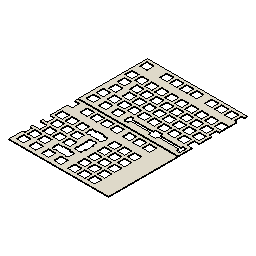
plate - F3D (Autodesk Fusion 360 design; units mm, degrees)
Autodesk Fusion 360 part; units mm, degrees
note: some values were not read from the file. Chosen so that the rebuilt part matches the saved one: which bodies a step acts on.
(part 1 of 3)
sketch "plate-2026-02-23T17_51_34.543Z" plane through (0, 0, 0) normal (0, 1, 0) x (1, 0, 0)
  line L0 (3.025, -2.525) -> (16.025, -2.525)
  line L1 (3.025, -16.525) -> (16.025, -16.525)
  line L2 (2.525, -3.025) -> (2.525, -16.025)
  line L3 (16.525, -3.025) -> (16.525, -16.025)
  arc A0 (3.025, -2.525) -> (2.525, -3.025) centre (3.025, -3.025) ccw
  arc A1 (16.525, -3.025) -> (16.025, -2.525) centre (16.025, -3.025) ccw
  arc A2 (2.525, -16.025) -> (3.025, -16.525) centre (3.025, -16.025) ccw
  arc A3 (16.025, -16.525) -> (16.525, -16.025) centre (16.025, -16.025) ccw
  line L4 (41.125, -2.525) -> (54.125, -2.525)
  line L5 (41.125, -16.525) -> (54.125, -16.525)
  line L6 (40.625, -3.025) -> (40.625, -16.025)
  line L7 (54.625, -3.025) -> (54.625, -16.025)
  arc A4 (41.125, -2.525) -> (40.625, -3.025) centre (41.125, -3.025) ccw
  arc A5 (54.625, -3.025) -> (54.125, -2.525) centre (54.125, -3.025) ccw
  arc A6 (40.625, -16.025) -> (41.125, -16.525) centre (41.125, -16.025) ccw
  arc A7 (54.125, -16.525) -> (54.625, -16.025) centre (54.125, -16.025) ccw
  line L8 (60.175, -2.525) -> (73.175, -2.525)
  line L9 (60.175, -16.525) -> (73.175, -16.525)
  line L10 (59.675, -3.025) -> (59.675, -16.025)
  line L11 (73.675, -3.025) -> (73.675, -16.025)
  arc A8 (60.175, -2.525) -> (59.675, -3.025) centre (60.175, -3.025) ccw
  arc A9 (73.675, -3.025) -> (73.175, -2.525) centre (73.175, -3.025) ccw
  arc A10 (59.675, -16.025) -> (60.175, -16.525) centre (60.175, -16.025) ccw
  arc A11 (73.175, -16.525) -> (73.675, -16.025) centre (73.175, -16.025) ccw
  line L12 (79.225, -2.525) -> (92.225, -2.525)
  line L13 (79.225, -16.525) -> (92.225, -16.525)
  line L14 (78.725, -3.025) -> (78.725, -16.025)
  line L15 (92.725, -3.025) -> (92.725, -16.025)
  arc A12 (79.225, -2.525) -> (78.725, -3.025) centre (79.225, -3.025) ccw
  arc A13 (92.725, -3.025) -> (92.225, -2.525) centre (92.225, -3.025) ccw
  arc A14 (78.725, -16.025) -> (79.225, -16.525) centre (79.225, -16.025) ccw
  arc A15 (92.225, -16.525) -> (92.725, -16.025) centre (92.225, -16.025) ccw
  line L16 (98.275, -2.525) -> (111.275, -2.525)
  line L17 (98.275, -16.525) -> (111.275, -16.525)
  line L18 (97.775, -3.025) -> (97.775, -16.025)
  line L19 (111.775, -3.025) -> (111.775, -16.025)
  arc A16 (98.275, -2.525) -> (97.775, -3.025) centre (98.275, -3.025) ccw
  arc A17 (111.775, -3.025) -> (111.275, -2.525) centre (111.275, -3.025) ccw
  arc A18 (97.775, -16.025) -> (98.275, -16.525) centre (98.275, -16.025) ccw
  arc A19 (111.275, -16.525) -> (111.775, -16.025) centre (111.275, -16.025) ccw
  line L20 (126.85, -2.525) -> (139.85, -2.525)
  line L21 (126.85, -16.525) -> (139.85, -16.525)
  line L22 (126.35, -3.025) -> (126.35, -16.025)
  line L23 (140.35, -3.025) -> (140.35, -16.025)
  arc A20 (126.85, -2.525) -> (126.35, -3.025) centre (126.85, -3.025) ccw
  arc A21 (140.35, -3.025) -> (139.85, -2.525) centre (139.85, -3.025) ccw
  arc A22 (126.35, -16.025) -> (126.85, -16.525) centre (126.85, -16.025) ccw
  arc A23 (139.85, -16.525) -> (140.35, -16.025) centre (139.85, -16.025) ccw
  line L24 (145.9, -2.525) -> (158.9, -2.525)
  line L25 (145.9, -16.525) -> (158.9, -16.525)
  line L26 (145.4, -3.025) -> (145.4, -16.025)
  line L27 (159.4, -3.025) -> (159.4, -16.025)
  arc A24 (145.9, -2.525) -> (145.4, -3.025) centre (145.9, -3.025) ccw
  arc A25 (159.4, -3.025) -> (158.9, -2.525) centre (158.9, -3.025) ccw
  arc A26 (145.4, -16.025) -> (145.9, -16.525) centre (145.9, -16.025) ccw
  arc A27 (158.9, -16.525) -> (159.4, -16.025) centre (158.9, -16.025) ccw
  line L28 (164.95, -2.525) -> (177.95, -2.525)
  line L29 (164.95, -16.525) -> (177.95, -16.525)
  line L30 (164.45, -3.025) -> (164.45, -16.025)
  line L31 (178.45, -3.025) -> (178.45, -16.025)
  arc A28 (164.95, -2.525) -> (164.45, -3.025) centre (164.95, -3.025) ccw
  arc A29 (178.45, -3.025) -> (177.95, -2.525) centre (177.95, -3.025) ccw
  arc A30 (164.45, -16.025) -> (164.95, -16.525) centre (164.95, -16.025) ccw
  arc A31 (177.95, -16.525) -> (178.45, -16.025) centre (177.95, -16.025) ccw
  line L32 (184, -2.525) -> (197, -2.525)
  line L33 (184, -16.525) -> (197, -16.525)
  line L34 (183.5, -3.025) -> (183.5, -16.025)
  line L35 (197.5, -3.025) -> (197.5, -16.025)
  arc A32 (184, -2.525) -> (183.5, -3.025) centre (184, -3.025) ccw
  arc A33 (197.5, -3.025) -> (197, -2.525) centre (197, -3.025) ccw
  arc A34 (183.5, -16.025) -> (184, -16.525) centre (184, -16.025) ccw
  arc A35 (197, -16.525) -> (197.5, -16.025) centre (197, -16.025) ccw
  line L36 (212.575, -2.525) -> (225.575, -2.525)
  line L37 (212.575, -16.525) -> (225.575, -16.525)
  line L38 (212.075, -3.025) -> (212.075, -16.025)
  line L39 (226.075, -3.025) -> (226.075, -16.025)
  arc A36 (212.575, -2.525) -> (212.075, -3.025) centre (212.575, -3.025) ccw
  arc A37 (226.075, -3.025) -> (225.575, -2.525) centre (225.575, -3.025) ccw
  arc A38 (212.075, -16.025) -> (212.575, -16.525) centre (212.575, -16.025) ccw
  arc A39 (225.575, -16.525) -> (226.075, -16.025) centre (225.575, -16.025) ccw
  line L40 (231.625, -2.525) -> (244.625, -2.525)
  line L41 (231.625, -16.525) -> (244.625, -16.525)
  line L42 (231.125, -3.025) -> (231.125, -16.025)
  line L43 (245.125, -3.025) -> (245.125, -16.025)
  arc A40 (231.625, -2.525) -> (231.125, -3.025) centre (231.625, -3.025) ccw
  arc A41 (245.125, -3.025) -> (244.625, -2.525) centre (244.625, -3.025) ccw
  arc A42 (231.125, -16.025) -> (231.625, -16.525) centre (231.625, -16.025) ccw
  arc A43 (244.625, -16.525) -> (245.125, -16.025) centre (244.625, -16.025) ccw
  line L44 (250.675, -2.525) -> (263.675, -2.525)
  line L45 (250.675, -16.525) -> (263.675, -16.525)
  line L46 (250.175, -3.025) -> (250.175, -16.025)
  line L47 (264.175, -3.025) -> (264.175, -16.025)
  arc A44 (250.675, -2.525) -> (250.175, -3.025) centre (250.675, -3.025) ccw
  arc A45 (264.175, -3.025) -> (263.675, -2.525) centre (263.675, -3.025) ccw
  arc A46 (250.175, -16.025) -> (250.675, -16.525) centre (250.675, -16.025) ccw
  arc A47 (263.675, -16.525) -> (264.175, -16.025) centre (263.675, -16.025) ccw
  line L48 (269.725, -2.525) -> (282.725, -2.525)
  line L49 (269.725, -16.525) -> (282.725, -16.525)
  line L50 (269.225, -3.025) -> (269.225, -16.025)
  line L51 (283.225, -3.025) -> (283.225, -16.025)
  arc A48 (269.725, -2.525) -> (269.225, -3.025) centre (269.725, -3.025) ccw
  arc A49 (283.225, -3.025) -> (282.725, -2.525) centre (282.725, -3.025) ccw
  arc A50 (269.225, -16.025) -> (269.725, -16.525) centre (269.725, -16.025) ccw
  arc A51 (282.725, -16.525) -> (283.225, -16.025) centre (282.725, -16.025) ccw
  line L52 (293.5375, -2.525) -> (306.5375, -2.525)
  line L53 (293.5375, -16.525) -> (306.5375, -16.525)
  line L54 (293.0375, -3.025) -> (293.0375, -16.025)
  line L55 (307.0375, -3.025) -> (307.0375, -16.025)
  arc A52 (293.5375, -2.525) -> (293.0375, -3.025) centre (293.5375, -3.025) ccw
  arc A53 (307.0375, -3.025) -> (306.5375, -2.525) centre (306.5375, -3.025) ccw
  arc A54 (293.0375, -16.025) -> (293.5375, -16.525) centre (293.5375, -16.025) ccw
  arc A55 (306.5375, -16.525) -> (307.0375, -16.025) centre (306.5375, -16.025) ccw
  line L56 (312.5875, -2.525) -> (325.5875, -2.525)
  line L57 (312.5875, -16.525) -> (325.5875, -16.525)
  line L58 (312.0875, -3.025) -> (312.0875, -16.025)
  line L59 (326.0875, -3.025) -> (326.0875, -16.025)
  arc A56 (312.5875, -2.525) -> (312.0875, -3.025) centre (312.5875, -3.025) ccw
  arc A57 (326.0875, -3.025) -> (325.5875, -2.525) centre (325.5875, -3.025) ccw
  arc A58 (312.0875, -16.025) -> (312.5875, -16.525) centre (312.5875, -16.025) ccw
  arc A59 (325.5875, -16.525) -> (326.0875, -16.025) centre (325.5875, -16.025) ccw
  line L60 (331.6375, -2.525) -> (344.6375, -2.525)
  line L61 (331.6375, -16.525) -> (344.6375, -16.525)
  line L62 (331.1375, -3.025) -> (331.1375, -16.025)
  line L63 (345.1375, -3.025) -> (345.1375, -16.025)
  arc A60 (331.6375, -2.525) -> (331.1375, -3.025) centre (331.6375, -3.025) ccw
  arc A61 (345.1375, -3.025) -> (344.6375, -2.525) centre (344.6375, -3.025) ccw
  arc A62 (331.1375, -16.025) -> (331.6375, -16.525) centre (331.6375, -16.025) ccw
  arc A63 (344.6375, -16.525) -> (345.1375, -16.025) centre (344.6375, -16.025) ccw
  line L64 (3.025, -31.1) -> (16.025, -31.1)
  line L65 (3.025, -45.1) -> (16.025, -45.1)
  line L66 (2.525, -31.6) -> (2.525, -44.6)
  line L67 (16.525, -31.6) -> (16.525, -44.6)
  arc A64 (3.025, -31.1) -> (2.525, -31.6) centre (3.025, -31.6) ccw
  arc A65 (16.525, -31.6) -> (16.025, -31.1) centre (16.025, -31.6) ccw
  arc A66 (2.525, -44.6) -> (3.025, -45.1) centre (3.025, -44.6) ccw
  arc A67 (16.025, -45.1) -> (16.525, -44.6) centre (16.025, -44.6) ccw
  line L68 (22.075, -31.1) -> (35.075, -31.1)
  line L69 (22.075, -45.1) -> (35.075, -45.1)
  line L70 (21.575, -31.6) -> (21.575, -44.6)
  line L71 (35.575, -31.6) -> (35.575, -44.6)
  arc A68 (22.075, -31.1) -> (21.575, -31.6) centre (22.075, -31.6) ccw
  arc A69 (35.575, -31.6) -> (35.075, -31.1) centre (35.075, -31.6) ccw
  arc A70 (21.575, -44.6) -> (22.075, -45.1) centre (22.075, -44.6) ccw
  arc A71 (35.075, -45.1) -> (35.575, -44.6) centre (35.075, -44.6) ccw
  line L72 (41.125, -31.1) -> (54.125, -31.1)
  line L73 (41.125, -45.1) -> (54.125, -45.1)
  line L74 (40.625, -31.6) -> (40.625, -44.6)
  line L75 (54.625, -31.6) -> (54.625, -44.6)
  arc A72 (41.125, -31.1) -> (40.625, -31.6) centre (41.125, -31.6) ccw
  arc A73 (54.625, -31.6) -> (54.125, -31.1) centre (54.125, -31.6) ccw
  arc A74 (40.625, -44.6) -> (41.125, -45.1) centre (41.125, -44.6) ccw
  arc A75 (54.125, -45.1) -> (54.625, -44.6) centre (54.125, -44.6) ccw
  line L76 (60.175, -31.1) -> (73.175, -31.1)
  line L77 (60.175, -45.1) -> (73.175, -45.1)
  line L78 (59.675, -31.6) -> (59.675, -44.6)
  line L79 (73.675, -31.6) -> (73.675, -44.6)
  arc A76 (60.175, -31.1) -> (59.675, -31.6) centre (60.175, -31.6) ccw
  arc A77 (73.675, -31.6) -> (73.175, -31.1) centre (73.175, -31.6) ccw
  arc A78 (59.675, -44.6) -> (60.175, -45.1) centre (60.175, -44.6) ccw
  arc A79 (73.175, -45.1) -> (73.675, -44.6) centre (73.175, -44.6) ccw
  line L80 (79.225, -31.1) -> (92.225, -31.1)
  line L81 (79.225, -45.1) -> (92.225, -45.1)
  line L82 (78.725, -31.6) -> (78.725, -44.6)
  line L83 (92.725, -31.6) -> (92.725, -44.6)
  arc A80 (79.225, -31.1) -> (78.725, -31.6) centre (79.225, -31.6) ccw
  arc A81 (92.725, -31.6) -> (92.225, -31.1) centre (92.225, -31.6) ccw
  arc A82 (78.725, -44.6) -> (79.225, -45.1) centre (79.225, -44.6) ccw
  arc A83 (92.225, -45.1) -> (92.725, -44.6) centre (92.225, -44.6) ccw
  line L84 (98.275, -31.1) -> (111.275, -31.1)
  line L85 (98.275, -45.1) -> (111.275, -45.1)
  line L86 (97.775, -31.6) -> (97.775, -44.6)
  line L87 (111.775, -31.6) -> (111.775, -44.6)
  arc A84 (98.275, -31.1) -> (97.775, -31.6) centre (98.275, -31.6) ccw
  arc A85 (111.775, -31.6) -> (111.275, -31.1) centre (111.275, -31.6) ccw
  arc A86 (97.775, -44.6) -> (98.275, -45.1) centre (98.275, -44.6) ccw
  arc A87 (111.275, -45.1) -> (111.775, -44.6) centre (111.275, -44.6) ccw
  line L88 (117.325, -31.1) -> (130.325, -31.1)
  line L89 (117.325, -45.1) -> (130.325, -45.1)
  line L90 (116.825, -31.6) -> (116.825, -44.6)
  line L91 (130.825, -31.6) -> (130.825, -44.6)
  arc A88 (117.325, -31.1) -> (116.825, -31.6) centre (117.325, -31.6) ccw
  arc A89 (130.825, -31.6) -> (130.325, -31.1) centre (130.325, -31.6) ccw
  arc A90 (116.825, -44.6) -> (117.325, -45.1) centre (117.325, -44.6) ccw
  arc A91 (130.325, -45.1) -> (130.825, -44.6) centre (130.325, -44.6) ccw
  line L92 (136.375, -31.1) -> (149.375, -31.1)
  line L93 (136.375, -45.1) -> (149.375, -45.1)
  line L94 (135.875, -31.6) -> (135.875, -44.6)
  line L95 (149.875, -31.6) -> (149.875, -44.6)
  arc A92 (136.375, -31.1) -> (135.875, -31.6) centre (136.375, -31.6) ccw
  arc A93 (149.875, -31.6) -> (149.375, -31.1) centre (149.375, -31.6) ccw
  arc A94 (135.875, -44.6) -> (136.375, -45.1) centre (136.375, -44.6) ccw
  arc A95 (149.375, -45.1) -> (149.875, -44.6) centre (149.375, -44.6) ccw
  line L96 (155.425, -31.1) -> (168.425, -31.1)
  line L97 (155.425, -45.1) -> (168.425, -45.1)
  line L98 (154.925, -31.6) -> (154.925, -44.6)
  line L99 (168.925, -31.6) -> (168.925, -44.6)
  arc A96 (155.425, -31.1) -> (154.925, -31.6) centre (155.425, -31.6) ccw
  arc A97 (168.925, -31.6) -> (168.425, -31.1) centre (168.425, -31.6) ccw
  arc A98 (154.925, -44.6) -> (155.425, -45.1) centre (155.425, -44.6) ccw
  arc A99 (168.425, -45.1) -> (168.925, -44.6) centre (168.425, -44.6) ccw
  line L100 (174.475, -31.1) -> (187.475, -31.1)
  line L101 (174.475, -45.1) -> (187.475, -45.1)
  line L102 (173.975, -31.6) -> (173.975, -44.6)
  line L103 (187.975, -31.6) -> (187.975, -44.6)
  arc A100 (174.475, -31.1) -> (173.975, -31.6) centre (174.475, -31.6) ccw
  arc A101 (187.975, -31.6) -> (187.475, -31.1) centre (187.475, -31.6) ccw
  arc A102 (173.975, -44.6) -> (174.475, -45.1) centre (174.475, -44.6) ccw
  arc A103 (187.475, -45.1) -> (187.975, -44.6) centre (187.475, -44.6) ccw
  line L104 (193.525, -31.1) -> (206.525, -31.1)
  line L105 (193.525, -45.1) -> (206.525, -45.1)
  line L106 (193.025, -31.6) -> (193.025, -44.6)
  line L107 (207.025, -31.6) -> (207.025, -44.6)
  arc A104 (193.525, -31.1) -> (193.025, -31.6) centre (193.525, -31.6) ccw
  arc A105 (207.025, -31.6) -> (206.525, -31.1) centre (206.525, -31.6) ccw
  arc A106 (193.025, -44.6) -> (193.525, -45.1) centre (193.525, -44.6) ccw
  arc A107 (206.525, -45.1) -> (207.025, -44.6) centre (206.525, -44.6) ccw
  line L108 (212.575, -31.1) -> (225.575, -31.1)
  line L109 (212.575, -45.1) -> (225.575, -45.1)
  line L110 (212.075, -31.6) -> (212.075, -44.6)
  line L111 (226.075, -31.6) -> (226.075, -44.6)
  arc A108 (212.575, -31.1) -> (212.075, -31.6) centre (212.575, -31.6) ccw
  arc A109 (226.075, -31.6) -> (225.575, -31.1) centre (225.575, -31.6) ccw
  arc A110 (212.075, -44.6) -> (212.575, -45.1) centre (212.575, -44.6) ccw
  arc A111 (225.575, -45.1) -> (226.075, -44.6) centre (225.575, -44.6) ccw
  line L112 (231.625, -31.1) -> (244.625, -31.1)
  line L113 (231.625, -45.1) -> (244.625, -45.1)
  line L114 (231.125, -31.6) -> (231.125, -44.6)
  line L115 (245.125, -31.6) -> (245.125, -44.6)
  arc A112 (231.625, -31.1) -> (231.125, -31.6) centre (231.625, -31.6) ccw
  arc A113 (245.125, -31.6) -> (244.625, -31.1) centre (244.625, -31.6) ccw
  arc A114 (231.125, -44.6) -> (231.625, -45.1) centre (231.625, -44.6) ccw
  arc A115 (244.625, -45.1) -> (245.125, -44.6) centre (244.625, -44.6) ccw
  line L116 (260.2, -31.1) -> (273.2, -31.1)
  line L117 (260.2, -45.1) -> (273.2, -45.1)
  line L118 (259.7, -31.6) -> (259.7, -44.6)
  line L119 (273.7, -31.6) -> (273.7, -44.6)
  arc A116 (260.2, -31.1) -> (259.7, -31.6) centre (260.2, -31.6) ccw
  arc A117 (273.7, -31.6) -> (273.2, -31.1) centre (273.2, -31.6) ccw
  arc A118 (259.7, -44.6) -> (260.2, -45.1) centre (260.2, -44.6) ccw
  arc A119 (273.2, -45.1) -> (273.7, -44.6) centre (273.2, -44.6) ccw
  line L120 (251.9346, -32.4104) -> (257.5894, -32.4104)
  line L121 (258.0894, -32.9104) -> (258.0894, -33.2232)
  line L122 (258.0894, -33.2232) -> (266.7, -33.2232)
  line L123 (266.7, -43.9166) -> (258.5894, -43.9166)
  line L124 (258.0894, -44.4166) -> (258.0894, -44.704)
  line L125 (258.0894, -44.704) -> (256.786, -44.704)
  line L126 (256.286, -45.204) -> (256.286, -45.3724)
  line L127 (255.786, -45.8724) -> (253.738, -45.8724)
  line L128 (253.238, -45.3724) -> (253.238, -45.204)
  line L129 (252.738, -44.704) -> (251.9346, -44.704)
  line L130 (251.4346, -44.204) -> (251.4346, -39.108)
  line L131 (250.9346, -38.608) -> (250.571, -38.608)
  line L132 (250.571, -38.608) -> (250.571, -36.314)
  line L133 (251.071, -35.814) -> (251.4346, -35.814)
  line L134 (251.4346, -35.814) -> (251.4346, -32.9104)
  arc A120 (258.0894, -32.9104) -> (257.5894, -32.4104) centre (257.5894, -32.9104) ccw
  arc A121 (258.5894, -43.9166) -> (258.0894, -44.4166) centre (258.5894, -44.4166) ccw
  arc A122 (256.786, -44.704) -> (256.286, -45.204) centre (256.786, -45.204) ccw
  arc A123 (255.786, -45.8724) -> (256.286, -45.3724) centre (255.786, -45.3724) ccw
  arc A124 (253.238, -45.3724) -> (253.738, -45.8724) centre (253.738, -45.3724) ccw
  arc A125 (253.238, -45.204) -> (252.738, -44.704) centre (252.738, -45.204) ccw
  arc A126 (251.4346, -44.204) -> (251.9346, -44.704) centre (251.9346, -44.204) ccw
  arc A127 (251.4346, -39.108) -> (250.9346, -38.608) centre (250.9346, -39.108) ccw
  arc A128 (251.071, -35.814) -> (250.571, -36.314) centre (251.071, -36.314) ccw
  arc A129 (251.9346, -32.4104) -> (251.4346, -32.9104) centre (251.9346, -32.9104) ccw
  line L135 (281.4654, -32.4104) -> (275.8106, -32.4104)
  line L136 (275.3106, -32.9104) -> (275.3106, -33.2232)
  line L137 (275.3106, -33.2232) -> (266.7, -33.2232)
  line L138 (266.7, -43.9166) -> (274.8106, -43.9166)
  line L139 (275.3106, -44.4166) -> (275.3106, -44.704)
  line L140 (275.3106, -44.704) -> (276.614, -44.704)
  line L141 (277.114, -45.204) -> (277.114, -45.3724)
  line L142 (277.614, -45.8724) -> (279.662, -45.8724)
  line L143 (280.162, -45.3724) -> (280.162, -45.204)
  line L144 (280.662, -44.704) -> (281.4654, -44.704)
  line L145 (281.9654, -44.204) -> (281.9654, -39.108)
  line L146 (282.4654, -38.608) -> (282.829, -38.608)
  line L147 (282.829, -38.608) -> (282.829, -36.314)
  line L148 (282.329, -35.814) -> (281.9654, -35.814)
  line L149 (281.9654, -35.814) -> (281.9654, -32.9104)
  arc A130 (275.8106, -32.4104) -> (275.3106, -32.9104) centre (275.8106, -32.9104) ccw
  arc A131 (275.3106, -44.4166) -> (274.8106, -43.9166) centre (274.8106, -44.4166) ccw
  arc A132 (277.114, -45.204) -> (276.614, -44.704) centre (276.614, -45.204) ccw
  arc A133 (277.114, -45.3724) -> (277.614, -45.8724) centre (277.614, -45.3724) ccw
  arc A134 (279.662, -45.8724) -> (280.162, -45.3724) centre (279.662, -45.3724) ccw
  arc A135 (280.662, -44.704) -> (280.162, -45.204) centre (280.662, -45.204) ccw
  arc A136 (281.4654, -44.704) -> (281.9654, -44.204) centre (281.4654, -44.204) ccw
  arc A137 (282.4654, -38.608) -> (281.9654, -39.108) centre (282.4654, -39.108) ccw
  arc A138 (282.829, -36.314) -> (282.329, -35.814) centre (282.329, -36.314) ccw
  arc A139 (281.9654, -32.9104) -> (281.4654, -32.4104) centre (281.4654, -32.9104) ccw
  line L150 (293.5375, -31.1) -> (306.5375, -31.1)
  line L151 (293.5375, -45.1) -> (306.5375, -45.1)
  line L152 (293.0375, -31.6) -> (293.0375, -44.6)
  line L153 (307.0375, -31.6) -> (307.0375, -44.6)
  arc A140 (293.5375, -31.1) -> (293.0375, -31.6) centre (293.5375, -31.6) ccw
  arc A141 (307.0375, -31.6) -> (306.5375, -31.1) centre (306.5375, -31.6) ccw
  arc A142 (293.0375, -44.6) -> (293.5375, -45.1) centre (293.5375, -44.6) ccw
  arc A143 (306.5375, -45.1) -> (307.0375, -44.6) centre (306.5375, -44.6) ccw
  line L154 (312.5875, -31.1) -> (325.5875, -31.1)
  line L155 (312.5875, -45.1) -> (325.5875, -45.1)
  line L156 (312.0875, -31.6) -> (312.0875, -44.6)
  line L157 (326.0875, -31.6) -> (326.0875, -44.6)
  arc A144 (312.5875, -31.1) -> (312.0875, -31.6) centre (312.5875, -31.6) ccw
  arc A145 (326.0875, -31.6) -> (325.5875, -31.1) centre (325.5875, -31.6) ccw
  arc A146 (312.0875, -44.6) -> (312.5875, -45.1) centre (312.5875, -44.6) ccw
  arc A147 (325.5875, -45.1) -> (326.0875, -44.6) centre (325.5875, -44.6) ccw
  line L158 (331.6375, -31.1) -> (344.6375, -31.1)
  line L159 (331.6375, -45.1) -> (344.6375, -45.1)
  line L160 (331.1375, -31.6) -> (331.1375, -44.6)
  line L161 (345.1375, -31.6) -> (345.1375, -44.6)
  arc A148 (331.6375, -31.1) -> (331.1375, -31.6) centre (331.6375, -31.6) ccw
  arc A149 (345.1375, -31.6) -> (344.6375, -31.1) centre (344.6375, -31.6) ccw
  arc A150 (331.1375, -44.6) -> (331.6375, -45.1) centre (331.6375, -44.6) ccw
  arc A151 (344.6375, -45.1) -> (345.1375, -44.6) centre (344.6375, -44.6) ccw
  line L162 (7.7875, -50.15) -> (20.7875, -50.15)
  line L163 (7.7875, -64.15) -> (20.7875, -64.15)
  line L164 (7.2875, -50.65) -> (7.2875, -63.65)
  line L165 (21.2875, -50.65) -> (21.2875, -63.65)
  arc A152 (7.7875, -50.15) -> (7.2875, -50.65) centre (7.7875, -50.65) ccw
  arc A153 (21.2875, -50.65) -> (20.7875, -50.15) centre (20.7875, -50.65) ccw
  arc A154 (7.2875, -63.65) -> (7.7875, -64.15) centre (7.7875, -63.65) ccw
  arc A155 (20.7875, -64.15) -> (21.2875, -63.65) centre (20.7875, -63.65) ccw
  line L166 (31.6, -50.15) -> (44.6, -50.15)
  line L167 (31.6, -64.15) -> (44.6, -64.15)
  line L168 (31.1, -50.65) -> (31.1, -63.65)
  line L169 (45.1, -50.65) -> (45.1, -63.65)
  arc A156 (31.6, -50.15) -> (31.1, -50.65) centre (31.6, -50.65) ccw
  arc A157 (45.1, -50.65) -> (44.6, -50.15) centre (44.6, -50.65) ccw
  arc A158 (31.1, -63.65) -> (31.6, -64.15) centre (31.6, -63.65) ccw
  arc A159 (44.6, -64.15) -> (45.1, -63.65) centre (44.6, -63.65) ccw
  line L170 (50.65, -50.15) -> (63.65, -50.15)
  line L171 (50.65, -64.15) -> (63.65, -64.15)
  line L172 (50.15, -50.65) -> (50.15, -63.65)
  line L173 (64.15, -50.65) -> (64.15, -63.65)
  arc A160 (50.65, -50.15) -> (50.15, -50.65) centre (50.65, -50.65) ccw
  arc A161 (64.15, -50.65) -> (63.65, -50.15) centre (63.65, -50.65) ccw
  arc A162 (50.15, -63.65) -> (50.65, -64.15) centre (50.65, -63.65) ccw
  arc A163 (63.65, -64.15) -> (64.15, -63.65) centre (63.65, -63.65) ccw
  line L174 (69.7, -50.15) -> (82.7, -50.15)
  line L175 (69.7, -64.15) -> (82.7, -64.15)
  line L176 (69.2, -50.65) -> (69.2, -63.65)
  line L177 (83.2, -50.65) -> (83.2, -63.65)
  arc A164 (69.7, -50.15) -> (69.2, -50.65) centre (69.7, -50.65) ccw
  arc A165 (83.2, -50.65) -> (82.7, -50.15) centre (82.7, -50.65) ccw
  arc A166 (69.2, -63.65) -> (69.7, -64.15) centre (69.7, -63.65) ccw
  arc A167 (82.7, -64.15) -> (83.2, -63.65) centre (82.7, -63.65) ccw
  line L178 (88.75, -50.15) -> (101.75, -50.15)
  line L179 (88.75, -64.15) -> (101.75, -64.15)
  line L180 (88.25, -50.65) -> (88.25, -63.65)
  line L181 (102.25, -50.65) -> (102.25, -63.65)
  arc A168 (88.75, -50.15) -> (88.25, -50.65) centre (88.75, -50.65) ccw
  arc A169 (102.25, -50.65) -> (101.75, -50.15) centre (101.75, -50.65) ccw
  arc A170 (88.25, -63.65) -> (88.75, -64.15) centre (88.75, -63.65) ccw
  arc A171 (101.75, -64.15) -> (102.25, -63.65) centre (101.75, -63.65) ccw
  line L182 (107.8, -50.15) -> (120.8, -50.15)
  line L183 (107.8, -64.15) -> (120.8, -64.15)
  line L184 (107.3, -50.65) -> (107.3, -63.65)
  line L185 (121.3, -50.65) -> (121.3, -63.65)
  arc A172 (107.8, -50.15) -> (107.3, -50.65) centre (107.8, -50.65) ccw
  arc A173 (121.3, -50.65) -> (120.8, -50.15) centre (120.8, -50.65) ccw
  arc A174 (107.3, -63.65) -> (107.8, -64.15) centre (107.8, -63.65) ccw
  arc A175 (120.8, -64.15) -> (121.3, -63.65) centre (120.8, -63.65) ccw
  line L186 (126.85, -50.15) -> (139.85, -50.15)
  line L187 (126.85, -64.15) -> (139.85, -64.15)
  line L188 (126.35, -50.65) -> (126.35, -63.65)
  line L189 (140.35, -50.65) -> (140.35, -63.65)
  arc A176 (126.85, -50.15) -> (126.35, -50.65) centre (126.85, -50.65) ccw
  arc A177 (140.35, -50.65) -> (139.85, -50.15) centre (139.85, -50.65) ccw
  arc A178 (126.35, -63.65) -> (126.85, -64.15) centre (126.85, -63.65) ccw
  arc A179 (139.85, -64.15) -> (140.35, -63.65) centre (139.85, -63.65) ccw
  line L190 (145.9, -50.15) -> (158.9, -50.15)
  line L191 (145.9, -64.15) -> (158.9, -64.15)
  line L192 (145.4, -50.65) -> (145.4, -63.65)
  line L193 (159.4, -50.65) -> (159.4, -63.65)
  arc A180 (145.9, -50.15) -> (145.4, -50.65) centre (145.9, -50.65) ccw
  arc A181 (159.4, -50.65) -> (158.9, -50.15) centre (158.9, -50.65) ccw
  arc A182 (145.4, -63.65) -> (145.9, -64.15) centre (145.9, -63.65) ccw
  arc A183 (158.9, -64.15) -> (159.4, -63.65) centre (158.9, -63.65) ccw
  line L194 (164.95, -50.15) -> (177.95, -50.15)
  line L195 (164.95, -64.15) -> (177.95, -64.15)
  line L196 (164.45, -50.65) -> (164.45, -63.65)
  line L197 (178.45, -50.65) -> (178.45, -63.65)
  arc A184 (164.95, -50.15) -> (164.45, -50.65) centre (164.95, -50.65) ccw
  arc A185 (178.45, -50.65) -> (177.95, -50.15) centre (177.95, -50.65) ccw
  arc A186 (164.45, -63.65) -> (164.95, -64.15) centre (164.95, -63.65) ccw
  arc A187 (177.95, -64.15) -> (178.45, -63.65) centre (177.95, -63.65) ccw
  line L198 (184, -50.15) -> (197, -50.15)
  line L199 (184, -64.15) -> (197, -64.15)
  line L200 (183.5, -50.65) -> (183.5, -63.65)
  line L201 (197.5, -50.65) -> (197.5, -63.65)
  arc A188 (184, -50.15) -> (183.5, -50.65) centre (184, -50.65) ccw
  arc A189 (197.5, -50.65) -> (197, -50.15) centre (197, -50.65) ccw
  arc A190 (183.5, -63.65) -> (184, -64.15) centre (184, -63.65) ccw
  arc A191 (197, -64.15) -> (197.5, -63.65) centre (197, -63.65) ccw
  line L202 (203.05, -50.15) -> (216.05, -50.15)
  line L203 (203.05, -64.15) -> (216.05, -64.15)
  line L204 (202.55, -50.65) -> (202.55, -63.65)
  line L205 (216.55, -50.65) -> (216.55, -63.65)
  arc A192 (203.05, -50.15) -> (202.55, -50.65) centre (203.05, -50.65) ccw
  arc A193 (216.55, -50.65) -> (216.05, -50.15) centre (216.05, -50.65) ccw
  arc A194 (202.55, -63.65) -> (203.05, -64.15) centre (203.05, -63.65) ccw
  arc A195 (216.05, -64.15) -> (216.55, -63.65) centre (216.05, -63.65) ccw
  line L206 (222.1, -50.15) -> (235.1, -50.15)
  line L207 (222.1, -64.15) -> (235.1, -64.15)
  line L208 (221.6, -50.65) -> (221.6, -63.65)
  line L209 (235.6, -50.65) -> (235.6, -63.65)
  arc A196 (222.1, -50.15) -> (221.6, -50.65) centre (222.1, -50.65) ccw
  arc A197 (235.6, -50.65) -> (235.1, -50.15) centre (235.1, -50.65) ccw
  arc A198 (221.6, -63.65) -> (222.1, -64.15) centre (222.1, -63.65) ccw
  arc A199 (235.1, -64.15) -> (235.6, -63.65) centre (235.1, -63.65) ccw
  line L210 (241.15, -50.15) -> (254.15, -50.15)
  line L211 (241.15, -64.15) -> (254.15, -64.15)
  line L212 (240.65, -50.65) -> (240.65, -63.65)
  line L213 (254.65, -50.65) -> (254.65, -63.65)
  arc A200 (241.15, -50.15) -> (240.65, -50.65) centre (241.15, -50.65) ccw
  arc A201 (254.65, -50.65) -> (254.15, -50.15) centre (254.15, -50.65) ccw
  arc A202 (240.65, -63.65) -> (241.15, -64.15) centre (241.15, -63.65) ccw
  arc A203 (254.15, -64.15) -> (254.65, -63.65) centre (254.15, -63.65) ccw
  line L214 (280.8438, -60.175) -> (280.8438, -73.175)
  line L215 (266.8438, -60.175) -> (266.8438, -73.175)
  line L216 (280.3438, -59.675) -> (267.3438, -59.675)
  line L217 (280.3438, -73.675) -> (267.3438, -73.675)
  arc A204 (280.8438, -60.175) -> (280.3438, -59.675) centre (280.3438, -60.175) ccw
  arc A205 (280.3438, -73.675) -> (280.8438, -73.175) centre (280.3438, -73.175) ccw
  arc A206 (267.3438, -59.675) -> (266.8438, -60.175) centre (267.3438, -60.175) ccw
  arc A207 (266.8438, -73.175) -> (267.3438, -73.675) centre (267.3438, -73.175) ccw
  line L218 (279.5333, -51.9096) -> (279.5333, -57.5644)
  line L219 (279.0333, -58.0644) -> (278.7206, -58.0644)
  line L220 (278.7206, -58.0644) -> (278.7206, -66.675)
  line L221 (268.0272, -66.675) -> (268.0272, -58.5644)
  line L222 (267.5272, -58.0644) -> (267.2398, -58.0644)
  line L223 (267.2398, -58.0644) -> (267.2398, -56.761)
  line L224 (266.7398, -56.261) -> (266.5713, -56.261)
  line L225 (266.0713, -55.761) -> (266.0713, -53.713)
  line L226 (266.5713, -53.213) -> (266.7398, -53.213)
  line L227 (267.2398, -52.713) -> (267.2398, -51.9096)
  line L228 (267.7398, -51.4096) -> (272.8358, -51.4096)
  line L229 (273.3358, -50.9096) -> (273.3358, -50.546)
  line L230 (273.3358, -50.546) -> (275.6298, -50.546)
  line L231 (276.1298, -51.046) -> (276.1298, -51.4096)
  line L232 (276.1298, -51.4096) -> (279.0333, -51.4096)
  arc A208 (279.0333, -58.0644) -> (279.5333, -57.5644) centre (279.0333, -57.5644) ccw
  arc A209 (268.0272, -58.5644) -> (267.5272, -58.0644) centre (267.5272, -58.5644) ccw
  arc A210 (267.2398, -56.761) -> (266.7398, -56.261) centre (266.7398, -56.761) ccw
  arc A211 (266.0713, -55.761) -> (266.5713, -56.261) centre (266.5713, -55.761) ccw
  arc A212 (266.5713, -53.213) -> (266.0713, -53.713) centre (266.5713, -53.713) ccw
  arc A213 (266.7398, -53.213) -> (267.2398, -52.713) centre (266.7398, -52.713) ccw
  arc A214 (267.7398, -51.4096) -> (267.2398, -51.9096) centre (267.7398, -51.9096) ccw
  arc A215 (272.8358, -51.4096) -> (273.3358, -50.9096) centre (272.8358, -50.9096) ccw
  arc A216 (276.1298, -51.046) -> (275.6298, -50.546) centre (275.6298, -51.046) ccw
  arc A217 (279.5333, -51.9096) -> (279.0333, -51.4096) centre (279.0333, -51.9096) ccw
  line L233 (279.5333, -81.4404) -> (279.5333, -75.7856)
  line L234 (279.0333, -75.2856) -> (278.7206, -75.2856)
  line L235 (278.7206, -75.2856) -> (278.7206, -66.675)
  line L236 (268.0272, -66.675) -> (268.0272, -74.7856)
  line L237 (267.5272, -75.2856) -> (267.2398, -75.2856)
  line L238 (267.2398, -75.2856) -> (267.2398, -76.589)
  line L239 (266.7398, -77.089) -> (266.5713, -77.089)
  line L240 (266.0713, -77.589) -> (266.0713, -79.637)
  line L241 (266.5713, -80.137) -> (266.7398, -80.137)
  line L242 (267.2398, -80.637) -> (267.2398, -81.4404)
  line L243 (267.7398, -81.9404) -> (272.8358, -81.9404)
  line L244 (273.3358, -82.4404) -> (273.3358, -82.804)
  line L245 (273.3358, -82.804) -> (275.6298, -82.804)
  line L246 (276.1298, -82.304) -> (276.1298, -81.9404)
  line L247 (276.1298, -81.9404) -> (279.0333, -81.9404)
  arc A218 (279.5333, -75.7856) -> (279.0333, -75.2856) centre (279.0333, -75.7856) ccw
  arc A219 (267.5272, -75.2856) -> (268.0272, -74.7856) centre (267.5272, -74.7856) ccw
  arc A220 (266.7398, -77.089) -> (267.2398, -76.589) centre (266.7398, -76.589) ccw
  arc A221 (266.5713, -77.089) -> (266.0713, -77.589) centre (266.5713, -77.589) ccw
  arc A222 (266.0713, -79.637) -> (266.5713, -80.137) centre (266.5713, -79.637) ccw
  arc A223 (267.2398, -80.637) -> (266.7398, -80.137) centre (266.7398, -80.637) ccw
  arc A224 (267.2398, -81.4404) -> (267.7398, -81.9404) centre (267.7398, -81.4404) ccw
  arc A225 (273.3358, -82.4404) -> (272.8358, -81.9404) centre (272.8358, -82.4404) ccw
  arc A226 (275.6298, -82.804) -> (276.1298, -82.304) centre (275.6298, -82.304) ccw
  arc A227 (279.0333, -81.9404) -> (279.5333, -81.4404) centre (279.0333, -81.4404) ccw
  line L248 (293.5375, -50.15) -> (306.5375, -50.15)
  line L249 (293.5375, -64.15) -> (306.5375, -64.15)
  line L250 (293.0375, -50.65) -> (293.0375, -63.65)
  line L251 (307.0375, -50.65) -> (307.0375, -63.65)
  arc A228 (293.5375, -50.15) -> (293.0375, -50.65) centre (293.5375, -50.65) ccw
  arc A229 (307.0375, -50.65) -> (306.5375, -50.15) centre (306.5375, -50.65) ccw
  arc A230 (293.0375, -63.65) -> (293.5375, -64.15) centre (293.5375, -63.65) ccw
  arc A231 (306.5375, -64.15) -> (307.0375, -63.65) centre (306.5375, -63.65) ccw
  line L252 (312.5875, -50.15) -> (325.5875, -50.15)
  line L253 (312.5875, -64.15) -> (325.5875, -64.15)
  line L254 (312.0875, -50.65) -> (312.0875, -63.65)
  line L255 (326.0875, -50.65) -> (326.0875, -63.65)
  arc A232 (312.5875, -50.15) -> (312.0875, -50.65) centre (312.5875, -50.65) ccw
  arc A233 (326.0875, -50.65) -> (325.5875, -50.15) centre (325.5875, -50.65) ccw
  arc A234 (312.0875, -63.65) -> (312.5875, -64.15) centre (312.5875, -63.65) ccw
  arc A235 (325.5875, -64.15) -> (326.0875, -63.65) centre (325.5875, -63.65) ccw
  line L256 (331.6375, -50.15) -> (344.6375, -50.15)
  line L257 (331.6375, -64.15) -> (344.6375, -64.15)
  line L258 (331.1375, -50.65) -> (331.1375, -63.65)
  line L259 (345.1375, -50.65) -> (345.1375, -63.65)
  arc A236 (331.6375, -50.15) -> (331.1375, -50.65) centre (331.6375, -50.65) ccw
  arc A237 (345.1375, -50.65) -> (344.6375, -50.15) centre (344.6375, -50.65) ccw
  arc A238 (331.1375, -63.65) -> (331.6375, -64.15) centre (331.6375, -63.65) ccw
  arc A239 (344.6375, -64.15) -> (345.1375, -63.65) centre (344.6375, -63.65) ccw
  line L260 (10.1687, -69.2) -> (23.1687, -69.2)
  line L261 (10.1687, -83.2) -> (23.1687, -83.2)
  line L262 (9.6687, -69.7) -> (9.6687, -82.7)
  line L263 (23.6687, -69.7) -> (23.6687, -82.7)
  arc A240 (10.1687, -69.2) -> (9.6688, -69.7) centre (10.1687, -69.7) ccw
  arc A241 (23.6687, -69.7) -> (23.1687, -69.2) centre (23.1687, -69.7) ccw
  arc A242 (9.6687, -82.7) -> (10.1687, -83.2) centre (10.1687, -82.7) ccw
  arc A243 (23.1687, -83.2) -> (23.6687, -82.7) centre (23.1687, -82.7) ccw
  line L264 (36.3625, -69.2) -> (49.3625, -69.2)
  line L265 (36.3625, -83.2) -> (49.3625, -83.2)
  line L266 (35.8625, -69.7) -> (35.8625, -82.7)
  line L267 (49.8625, -69.7) -> (49.8625, -82.7)
  arc A244 (36.3625, -69.2) -> (35.8625, -69.7) centre (36.3625, -69.7) ccw
  arc A245 (49.8625, -69.7) -> (49.3625, -69.2) centre (49.3625, -69.7) ccw
  arc A246 (35.8625, -82.7) -> (36.3625, -83.2) centre (36.3625, -82.7) ccw
  arc A247 (49.3625, -83.2) -> (49.8625, -82.7) centre (49.3625, -82.7) ccw
  line L268 (55.4125, -69.2) -> (68.4125, -69.2)
  line L269 (55.4125, -83.2) -> (68.4125, -83.2)
  line L270 (54.9125, -69.7) -> (54.9125, -82.7)
  line L271 (68.9125, -69.7) -> (68.9125, -82.7)
  arc A248 (55.4125, -69.2) -> (54.9125, -69.7) centre (55.4125, -69.7) ccw
  arc A249 (68.9125, -69.7) -> (68.4125, -69.2) centre (68.4125, -69.7) ccw
  arc A250 (54.9125, -82.7) -> (55.4125, -83.2) centre (55.4125, -82.7) ccw
  arc A251 (68.4125, -83.2) -> (68.9125, -82.7) centre (68.4125, -82.7) ccw
  line L272 (74.4625, -69.2) -> (87.4625, -69.2)
  line L273 (74.4625, -83.2) -> (87.4625, -83.2)
  line L274 (73.9625, -69.7) -> (73.9625, -82.7)
  line L275 (87.9625, -69.7) -> (87.9625, -82.7)
  arc A252 (74.4625, -69.2) -> (73.9625, -69.7) centre (74.4625, -69.7) ccw
  arc A253 (87.9625, -69.7) -> (87.4625, -69.2) centre (87.4625, -69.7) ccw
  arc A254 (73.9625, -82.7) -> (74.4625, -83.2) centre (74.4625, -82.7) ccw
  arc A255 (87.4625, -83.2) -> (87.9625, -82.7) centre (87.4625, -82.7) ccw
  line L276 (93.5125, -69.2) -> (106.5125, -69.2)
  line L277 (93.5125, -83.2) -> (106.5125, -83.2)
  line L278 (93.0125, -69.7) -> (93.0125, -82.7)
  line L279 (107.0125, -69.7) -> (107.0125, -82.7)
  arc A256 (93.5125, -69.2) -> (93.0125, -69.7) centre (93.5125, -69.7) ccw
  arc A257 (107.0125, -69.7) -> (106.5125, -69.2) centre (106.5125, -69.7) ccw
  arc A258 (93.0125, -82.7) -> (93.5125, -83.2) centre (93.5125, -82.7) ccw
  arc A259 (106.5125, -83.2) -> (107.0125, -82.7) centre (106.5125, -82.7) ccw
  line L280 (112.5625, -69.2) -> (125.5625, -69.2)
  line L281 (112.5625, -83.2) -> (125.5625, -83.2)
  line L282 (112.0625, -69.7) -> (112.0625, -82.7)
  line L283 (126.0625, -69.7) -> (126.0625, -82.7)
  arc A260 (112.5625, -69.2) -> (112.0625, -69.7) centre (112.5625, -69.7) ccw
  arc A261 (126.0625, -69.7) -> (125.5625, -69.2) centre (125.5625, -69.7) ccw
  arc A262 (112.0625, -82.7) -> (112.5625, -83.2) centre (112.5625, -82.7) ccw
  arc A263 (125.5625, -83.2) -> (126.0625, -82.7) centre (125.5625, -82.7) ccw
  line L284 (131.6125, -69.2) -> (144.6125, -69.2)
  line L285 (131.6125, -83.2) -> (144.6125, -83.2)
  line L286 (131.1125, -69.7) -> (131.1125, -82.7)
  line L287 (145.1125, -69.7) -> (145.1125, -82.7)
  arc A264 (131.6125, -69.2) -> (131.1125, -69.7) centre (131.6125, -69.7) ccw
  arc A265 (145.1125, -69.7) -> (144.6125, -69.2) centre (144.6125, -69.7) ccw
  arc A266 (131.1125, -82.7) -> (131.6125, -83.2) centre (131.6125, -82.7) ccw
  arc A267 (144.6125, -83.2) -> (145.1125, -82.7) centre (144.6125, -82.7) ccw
  line L288 (150.6625, -69.2) -> (163.6625, -69.2)
  line L289 (150.6625, -83.2) -> (163.6625, -83.2)
  line L290 (150.1625, -69.7) -> (150.1625, -82.7)
  line L291 (164.1625, -69.7) -> (164.1625, -82.7)
  arc A268 (150.6625, -69.2) -> (150.1625, -69.7) centre (150.6625, -69.7) ccw
  arc A269 (164.1625, -69.7) -> (163.6625, -69.2) centre (163.6625, -69.7) ccw
  arc A270 (150.1625, -82.7) -> (150.6625, -83.2) centre (150.6625, -82.7) ccw
  arc A271 (163.6625, -83.2) -> (164.1625, -82.7) centre (163.6625, -82.7) ccw
  line L292 (169.7125, -69.2) -> (182.7125, -69.2)
  line L293 (169.7125, -83.2) -> (182.7125, -83.2)
  line L294 (169.2125, -69.7) -> (169.2125, -82.7)
  line L295 (183.2125, -69.7) -> (183.2125, -82.7)
  arc A272 (169.7125, -69.2) -> (169.2125, -69.7) centre (169.7125, -69.7) ccw
  arc A273 (183.2125, -69.7) -> (182.7125, -69.2) centre (182.7125, -69.7) ccw
  arc A274 (169.2125, -82.7) -> (169.7125, -83.2) centre (169.7125, -82.7) ccw
  arc A275 (182.7125, -83.2) -> (183.2125, -82.7) centre (182.7125, -82.7) ccw
  line L296 (188.7625, -69.2) -> (201.7625, -69.2)
  line L297 (188.7625, -83.2) -> (201.7625, -83.2)
  line L298 (188.2625, -69.7) -> (188.2625, -82.7)
  line L299 (202.2625, -69.7) -> (202.2625, -82.7)
  arc A276 (188.7625, -69.2) -> (188.2625, -69.7) centre (188.7625, -69.7) ccw
  arc A277 (202.2625, -69.7) -> (201.7625, -69.2) centre (201.7625, -69.7) ccw
  arc A278 (188.2625, -82.7) -> (188.7625, -83.2) centre (188.7625, -82.7) ccw
  arc A279 (201.7625, -83.2) -> (202.2625, -82.7) centre (201.7625, -82.7) ccw
  line L300 (207.8125, -69.2) -> (220.8125, -69.2)
  line L301 (207.8125, -83.2) -> (220.8125, -83.2)
  line L302 (207.3125, -69.7) -> (207.3125, -82.7)
  line L303 (221.3125, -69.7) -> (221.3125, -82.7)
  arc A280 (207.8125, -69.2) -> (207.3125, -69.7) centre (207.8125, -69.7) ccw
  arc A281 (221.3125, -69.7) -> (220.8125, -69.2) centre (220.8125, -69.7) ccw
  arc A282 (207.3125, -82.7) -> (207.8125, -83.2) centre (207.8125, -82.7) ccw
  arc A283 (220.8125, -83.2) -> (221.3125, -82.7) centre (220.8125, -82.7) ccw
  line L304 (226.8625, -69.2) -> (239.8625, -69.2)
  line L305 (226.8625, -83.2) -> (239.8625, -83.2)
  line L306 (226.3625, -69.7) -> (226.3625, -82.7)
  line L307 (240.3625, -69.7) -> (240.3625, -82.7)
  arc A284 (226.8625, -69.2) -> (226.3625, -69.7) centre (226.8625, -69.7) ccw
  arc A285 (240.3625, -69.7) -> (239.8625, -69.2) centre (239.8625, -69.7) ccw
  arc A286 (226.3625, -82.7) -> (226.8625, -83.2) centre (226.8625, -82.7) ccw
  arc A287 (239.8625, -83.2) -> (240.3625, -82.7) centre (239.8625, -82.7) ccw
  line L308 (245.9125, -69.2) -> (258.9125, -69.2)
  line L309 (245.9125, -83.2) -> (258.9125, -83.2)
  line L310 (245.4125, -69.7) -> (245.4125, -82.7)
  line L311 (259.4125, -69.7) -> (259.4125, -82.7)
  arc A288 (245.9125, -69.2) -> (245.4125, -69.7) centre (245.9125, -69.7) ccw
  arc A289 (259.4125, -69.7) -> (258.9125, -69.2) centre (258.9125, -69.7) ccw
  arc A290 (245.4125, -82.7) -> (245.9125, -83.2) centre (245.9125, -82.7) ccw
  arc A291 (258.9125, -83.2) -> (259.4125, -82.7) centre (258.9125, -82.7) ccw
  line L312 (293.5375, -69.2) -> (306.5375, -69.2)
  line L313 (293.5375, -83.2) -> (306.5375, -83.2)
  line L314 (293.0375, -69.7) -> (293.0375, -82.7)
  line L315 (307.0375, -69.7) -> (307.0375, -82.7)
  arc A292 (293.5375, -69.2) -> (293.0375, -69.7) centre (293.5375, -69.7) ccw
  arc A293 (307.0375, -69.7) -> (306.5375, -69.2) centre (306.5375, -69.7) ccw
  arc A294 (293.0375, -82.7) -> (293.5375, -83.2) centre (293.5375, -82.7) ccw
  arc A295 (306.5375, -83.2) -> (307.0375, -82.7) centre (306.5375, -82.7) ccw
  line L316 (312.5875, -69.2) -> (325.5875, -69.2)
  line L317 (312.5875, -83.2) -> (325.5875, -83.2)
  line L318 (312.0875, -69.7) -> (312.0875, -82.7)
  line L319 (326.0875, -69.7) -> (326.0875, -82.7)
  arc A296 (312.5875, -69.2) -> (312.0875, -69.7) centre (312.5875, -69.7) ccw
  arc A297 (326.0875, -69.7) -> (325.5875, -69.2) centre (325.5875, -69.7) ccw
  arc A298 (312.0875, -82.7) -> (312.5875, -83.2) centre (312.5875, -82.7) ccw
  arc A299 (325.5875, -83.2) -> (326.0875, -82.7) centre (325.5875, -82.7) ccw
  line L320 (331.6375, -69.2) -> (344.6375, -69.2)
  line L321 (331.6375, -83.2) -> (344.6375, -83.2)
  line L322 (331.1375, -69.7) -> (331.1375, -82.7)
  line L323 (345.1375, -69.7) -> (345.1375, -82.7)
  arc A300 (331.6375, -69.2) -> (331.1375, -69.7) centre (331.6375, -69.7) ccw
  arc A301 (345.1375, -69.7) -> (344.6375, -69.2) centre (344.6375, -69.7) ccw
  arc A302 (331.1375, -82.7) -> (331.6375, -83.2) centre (331.6375, -82.7) ccw
  arc A303 (344.6375, -83.2) -> (345.1375, -82.7) centre (344.6375, -82.7) ccw
  line L324 (5.4062, -88.25) -> (18.4063, -88.25)
  line L325 (5.4062, -102.25) -> (18.4063, -102.25)
  line L326 (4.9062, -88.75) -> (4.9062, -101.75)
  line L327 (18.9062, -88.75) -> (18.9062, -101.75)
  arc A304 (5.4062, -88.25) -> (4.9063, -88.75) centre (5.4062, -88.75) ccw
  arc A305 (18.9062, -88.75) -> (18.4062, -88.25) centre (18.4062, -88.75) ccw
  arc A306 (4.9062, -101.75) -> (5.4062, -102.25) centre (5.4062, -101.75) ccw
  arc A307 (18.4062, -102.25) -> (18.9063, -101.75) centre (18.4062, -101.75) ccw
  line L328 (26.8375, -88.25) -> (39.8375, -88.25)
  line L329 (26.8375, -102.25) -> (39.8375, -102.25)
  line L330 (26.3375, -88.75) -> (26.3375, -101.75)
  line L331 (40.3375, -88.75) -> (40.3375, -101.75)
  arc A308 (26.8375, -88.25) -> (26.3375, -88.75) centre (26.8375, -88.75) ccw
  arc A309 (40.3375, -88.75) -> (39.8375, -88.25) centre (39.8375, -88.75) ccw
  arc A310 (26.3375, -101.75) -> (26.8375, -102.25) centre (26.8375, -101.75) ccw
  arc A311 (39.8375, -102.25) -> (40.3375, -101.75) centre (39.8375, -101.75) ccw
  line L332 (45.8875, -88.25) -> (58.8875, -88.25)
  line L333 (45.8875, -102.25) -> (58.8875, -102.25)
  line L334 (45.3875, -88.75) -> (45.3875, -101.75)
  line L335 (59.3875, -88.75) -> (59.3875, -101.75)
  arc A312 (45.8875, -88.25) -> (45.3875, -88.75) centre (45.8875, -88.75) ccw
  arc A313 (59.3875, -88.75) -> (58.8875, -88.25) centre (58.8875, -88.75) ccw
  arc A314 (45.3875, -101.75) -> (45.8875, -102.25) centre (45.8875, -101.75) ccw
  arc A315 (58.8875, -102.25) -> (59.3875, -101.75) centre (58.8875, -101.75) ccw
  line L336 (64.9375, -88.25) -> (77.9375, -88.25)
  line L337 (64.9375, -102.25) -> (77.9375, -102.25)
  line L338 (64.4375, -88.75) -> (64.4375, -101.75)
  line L339 (78.4375, -88.75) -> (78.4375, -101.75)
  arc A316 (64.9375, -88.25) -> (64.4375, -88.75) centre (64.9375, -88.75) ccw
  arc A317 (78.4375, -88.75) -> (77.9375, -88.25) centre (77.9375, -88.75) ccw
  arc A318 (64.4375, -101.75) -> (64.9375, -102.25) centre (64.9375, -101.75) ccw
  arc A319 (77.9375, -102.25) -> (78.4375, -101.75) centre (77.9375, -101.75) ccw
  line L340 (83.9875, -88.25) -> (96.9875, -88.25)
  line L341 (83.9875, -102.25) -> (96.9875, -102.25)
  line L342 (83.4875, -88.75) -> (83.4875, -101.75)
  line L343 (97.4875, -88.75) -> (97.4875, -101.75)
  arc A320 (83.9875, -88.25) -> (83.4875, -88.75) centre (83.9875, -88.75) ccw
  arc A321 (97.4875, -88.75) -> (96.9875, -88.25) centre (96.9875, -88.75) ccw
  arc A322 (83.4875, -101.75) -> (83.9875, -102.25) centre (83.9875, -101.75) ccw
  arc A323 (96.9875, -102.25) -> (97.4875, -101.75) centre (96.9875, -101.75) ccw
  line L344 (103.0375, -88.25) -> (116.0375, -88.25)
  line L345 (103.0375, -102.25) -> (116.0375, -102.25)
  line L346 (102.5375, -88.75) -> (102.5375, -101.75)
  line L347 (116.5375, -88.75) -> (116.5375, -101.75)
  arc A324 (103.0375, -88.25) -> (102.5375, -88.75) centre (103.0375, -88.75) ccw
  arc A325 (116.5375, -88.75) -> (116.0375, -88.25) centre (116.0375, -88.75) ccw
  arc A326 (102.5375, -101.75) -> (103.0375, -102.25) centre (103.0375, -101.75) ccw
  arc A327 (116.0375, -102.25) -> (116.5375, -101.75) centre (116.0375, -101.75) ccw
  line L348 (122.0875, -88.25) -> (135.0875, -88.25)
  line L349 (122.0875, -102.25) -> (135.0875, -102.25)
  line L350 (121.5875, -88.75) -> (121.5875, -101.75)
  line L351 (135.5875, -88.75) -> (135.5875, -101.75)
  arc A328 (122.0875, -88.25) -> (121.5875, -88.75) centre (122.0875, -88.75) ccw
  arc A329 (135.5875, -88.75) -> (135.0875, -88.25) centre (135.0875, -88.75) ccw
  arc A330 (121.5875, -101.75) -> (122.0875, -102.25) centre (122.0875, -101.75) ccw
  arc A331 (135.0875, -102.25) -> (135.5875, -101.75) centre (135.0875, -101.75) ccw
  line L352 (141.1375, -88.25) -> (154.1375, -88.25)
  line L353 (141.1375, -102.25) -> (154.1375, -102.25)
  line L354 (140.6375, -88.75) -> (140.6375, -101.75)
  line L355 (154.6375, -88.75) -> (154.6375, -101.75)
  arc A332 (141.1375, -88.25) -> (140.6375, -88.75) centre (141.1375, -88.75) ccw
  arc A333 (154.6375, -88.75) -> (154.1375, -88.25) centre (154.1375, -88.75) ccw
  arc A334 (140.6375, -101.75) -> (141.1375, -102.25) centre (141.1375, -101.75) ccw
  arc A335 (154.1375, -102.25) -> (154.6375, -101.75) centre (154.1375, -101.75) ccw
  line L356 (160.1875, -88.25) -> (173.1875, -88.25)
  line L357 (160.1875, -102.25) -> (173.1875, -102.25)
  line L358 (159.6875, -88.75) -> (159.6875, -101.75)
  line L359 (173.6875, -88.75) -> (173.6875, -101.75)
  arc A336 (160.1875, -88.25) -> (159.6875, -88.75) centre (160.1875, -88.75) ccw
  arc A337 (173.6875, -88.75) -> (173.1875, -88.25) centre (173.1875, -88.75) ccw
  arc A338 (159.6875, -101.75) -> (160.1875, -102.25) centre (160.1875, -101.75) ccw
  arc A339 (173.1875, -102.25) -> (173.6875, -101.75) centre (173.1875, -101.75) ccw
  line L360 (179.2375, -88.25) -> (192.2375, -88.25)
  line L361 (179.2375, -102.25) -> (192.2375, -102.25)
  line L362 (178.7375, -88.75) -> (178.7375, -101.75)
  line L363 (192.7375, -88.75) -> (192.7375, -101.75)
  arc A340 (179.2375, -88.25) -> (178.7375, -88.75) centre (179.2375, -88.75) ccw
  arc A341 (192.7375, -88.75) -> (192.2375, -88.25) centre (192.2375, -88.75) ccw
  arc A342 (178.7375, -101.75) -> (179.2375, -102.25) centre (179.2375, -101.75) ccw
  arc A343 (192.2375, -102.25) -> (192.7375, -101.75) centre (192.2375, -101.75) ccw
  line L364 (198.2875, -88.25) -> (211.2875, -88.25)
  line L365 (198.2875, -102.25) -> (211.2875, -102.25)
  line L366 (197.7875, -88.75) -> (197.7875, -101.75)
  line L367 (211.7875, -88.75) -> (211.7875, -101.75)
  arc A344 (198.2875, -88.25) -> (197.7875, -88.75) centre (198.2875, -88.75) ccw
  arc A345 (211.7875, -88.75) -> (211.2875, -88.25) centre (211.2875, -88.75) ccw
  arc A346 (197.7875, -101.75) -> (198.2875, -102.25) centre (198.2875, -101.75) ccw
  arc A347 (211.2875, -102.25) -> (211.7875, -101.75) centre (211.2875, -101.75) ccw
  line L368 (217.3375, -88.25) -> (230.3375, -88.25)
  line L369 (217.3375, -102.25) -> (230.3375, -102.25)
  line L370 (216.8375, -88.75) -> (216.8375, -101.75)
  line L371 (230.8375, -88.75) -> (230.8375, -101.75)
  arc A348 (217.3375, -88.25) -> (216.8375, -88.75) centre (217.3375, -88.75) ccw
  arc A349 (230.8375, -88.75) -> (230.3375, -88.25) centre (230.3375, -88.75) ccw
  arc A350 (216.8375, -101.75) -> (217.3375, -102.25) centre (217.3375, -101.75) ccw
  arc A351 (230.3375, -102.25) -> (230.8375, -101.75) centre (230.3375, -101.75) ccw
  line L372 (253.0563, -88.25) -> (266.0562, -88.25)
  line L373 (253.0563, -102.25) -> (266.0562, -102.25)
  line L374 (252.5563, -88.75) -> (252.5563, -101.75)
  line L375 (266.5562, -88.75) -> (266.5562, -101.75)
  arc A352 (253.0563, -88.25) -> (252.5563, -88.75) centre (253.0563, -88.75) ccw
  arc A353 (266.5562, -88.75) -> (266.0562, -88.25) centre (266.0562, -88.75) ccw
  arc A354 (252.5563, -101.75) -> (253.0563, -102.25) centre (253.0563, -101.75) ccw
  arc A355 (266.0562, -102.25) -> (266.5562, -101.75) centre (266.0562, -101.75) ccw
  line L376 (244.7909, -89.5604) -> (250.4457, -89.5604)
  line L377 (250.9457, -90.0604) -> (250.9457, -90.3732)
  line L378 (250.9457, -90.3732) -> (259.5562, -90.3732)
  line L379 (259.5562, -101.0666) -> (251.4457, -101.0666)
  line L380 (250.9457, -101.5666) -> (250.9457, -101.854)
  line L381 (250.9457, -101.854) -> (249.6422, -101.854)
  line L382 (249.1423, -102.354) -> (249.1423, -102.5224)
  line L383 (248.6423, -103.0224) -> (246.5942, -103.0224)
  line L384 (246.0943, -102.5224) -> (246.0943, -102.354)
  line L385 (245.5943, -101.854) -> (244.7909, -101.854)
  line L386 (244.2909, -101.354) -> (244.2909, -96.258)
  line L387 (243.7909, -95.758) -> (243.4273, -95.758)
  line L388 (243.4273, -95.758) -> (243.4273, -93.464)
  line L389 (243.9272, -92.964) -> (244.2909, -92.964)
  line L390 (244.2909, -92.964) -> (244.2909, -90.0604)
  arc A356 (250.9457, -90.0604) -> (250.4457, -89.5604) centre (250.4457, -90.0604) ccw
  arc A357 (251.4457, -101.0666) -> (250.9457, -101.5666) centre (251.4457, -101.5666) ccw
  arc A358 (249.6422, -101.854) -> (249.1422, -102.354) centre (249.6422, -102.354) ccw
  arc A359 (248.6423, -103.0224) -> (249.1423, -102.5224) centre (248.6423, -102.5224) ccw
  arc A360 (246.0943, -102.5224) -> (246.5942, -103.0224) centre (246.5942, -102.5224) ccw
  arc A361 (246.0943, -102.354) -> (245.5943, -101.854) centre (245.5943, -102.354) ccw
  arc A362 (244.2909, -101.354) -> (244.7909, -101.854) centre (244.7909, -101.354) ccw
  arc A363 (244.2909, -96.258) -> (243.7909, -95.758) centre (243.7909, -96.258) ccw
  arc A364 (243.9272, -92.964) -> (243.4272, -93.464) centre (243.9272, -93.464) ccw
  arc A365 (244.7909, -89.5604) -> (244.2909, -90.0604) centre (244.7909, -90.0604) ccw
  line L391 (274.3216, -89.5604) -> (268.6669, -89.5604)
  line L392 (268.1669, -90.0604) -> (268.1669, -90.3732)
  line L393 (268.1669, -90.3732) -> (259.5562, -90.3732)
  line L394 (259.5562, -101.0666) -> (267.6669, -101.0666)
  line L395 (268.1669, -101.5666) -> (268.1669, -101.854)
  line L396 (268.1669, -101.854) -> (269.4703, -101.854)
  line L397 (269.9703, -102.354) -> (269.9703, -102.5224)
  line L398 (270.4703, -103.0224) -> (272.5183, -103.0224)
  line L399 (273.0183, -102.5224) -> (273.0183, -102.354)
  line L400 (273.5183, -101.854) -> (274.3216, -101.854)
  line L401 (274.8216, -101.354) -> (274.8216, -96.258)
  line L402 (275.3216, -95.758) -> (275.6852, -95.758)
  line L403 (275.6852, -95.758) -> (275.6852, -93.464)